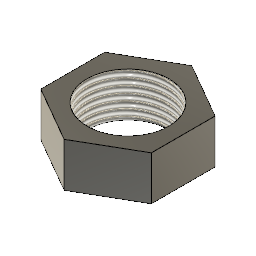
Semana3_Desafio6 v1 (Autodesk Fusion 360 design; units mm, degrees)
Autodesk Fusion 360 part; units mm, degrees
sketch "Sketch1" plane through (0, 0, 0) normal (0, 0, 1) x (1, 0, 0)
  line L0 (50, 28.8675) -> (0, 57.735)
  line L1 (0, 57.735) -> (-50, 28.8675)
  line L2 (-50, 28.8675) -> (-50, -28.8675)
  line L3 (-50, -28.8675) -> (0, -57.735)
  line L4 (0, -57.735) -> (50, -28.8675)
  line L5 (50, -28.8675) -> (50, 28.8675)
  dimension "d1" = 50
  measures "d1" distance of origin L5
extrude "Extrude1" add sketch "Sketch1" along normal mid plane 40
hole "Hole1" at (0, 0, 20) direction (0, 0, -1) diameter 73.905 end through all
thread "Thread1" "ISO Metric profile 80.0 M80x6 6H"
